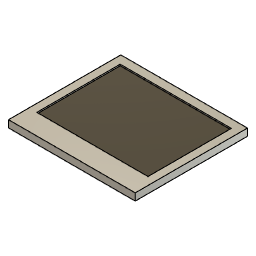
ER-TFT020-1 Display (Autodesk Fusion 360 design; units mm, degrees)
Autodesk Fusion 360 part; units mm, degrees
sketch "Sketch1" plane through (0, 0, 0) normal (0, 1, 0) x (1, 0, 0)
  line L0 (-10.4838, 8.3773) -> (36.0162, 8.3773)
  line L1 (36.0162, 8.3773) -> (36.0162, -32.8227)
  line L2 (36.0162, -32.8227) -> (-10.4838, -32.8227)
  line L3 (-10.4838, -32.8227) -> (-10.4838, 8.3773)
  dimension "d1" = 46.5
  dimension "d2" = 41.2
  constraint horizontal L0
  constraint vertical L1
  constraint horizontal L2
  constraint vertical L3
  measures "d1" distance of L0.start L0.end
  measures "d2" distance of L0.start L2.end
extrude "Extrude1" add sketch "Sketch1" along normal blind 2.62
sketch "Sketch2" plane through (0, 2.62, 0) normal (0, 1, 0) x (-1, 0, 0)
  line L0 (10.4838, 32.8227) -> (-36.0162, 32.8227)
  line L1 (-36.0162, 32.8227) -> (-36.0162, -8.3773)
  line L2 (-36.0162, -8.3773) -> (10.4838, -8.3773)
  line L3 (10.4838, -8.3773) -> (10.4838, 32.8227)
  line L4 (7.6338, -5.3073) -> (-33.1662, -5.3073)
  line L5 (-33.1662, -5.3073) -> (-33.1662, 25.2927)
  line L6 (-33.1662, 25.2927) -> (7.6338, 25.2927)
  line L7 (7.6338, 25.2927) -> (7.6338, -5.3073)
  line L8 (-12.7662, -8.3773) -> (-12.7662, 32.8227)
  dimension "d5" = 40.8
  dimension "d6" = 30.6
  dimension "d7" = 3.07
  constraint horizontal L4
  constraint vertical L5
  constraint horizontal L6
  constraint vertical L7
  constraint midpoint L2 L8.start
  constraint midpoint L0 L8.end
  constraint symmetric L5 L7 L8
  measures "d5" distance of L4.start L4.end
  measures "d6" distance of L4.end L5.end
  measures "d7" distance of L2 L4
extrude "Extrude2" cut sketch "Sketch2" against normal blind 0.5 contours L4 L5 L6 L8 | L4 L6 L7 L8
